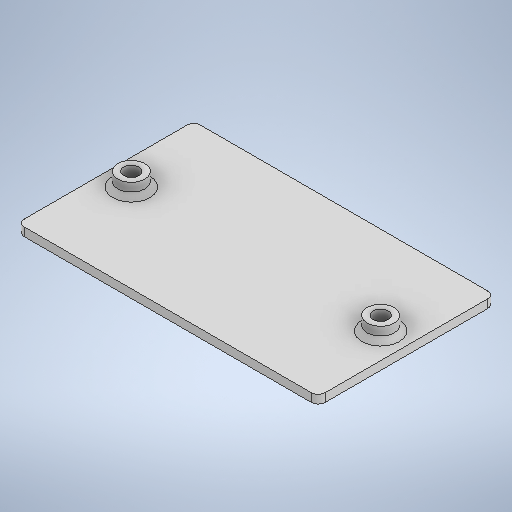
# Autodesk Inventor part: medium_backplate
Saved by Autodesk Inventor 2025.2 (Build 292293000, 293)
## iProperties
Created: 2025-04-21
Part Number: medium_backplate
Material: Generic
Document SubType Name: Modeling
Designer: osmon
Density: 1 g/cm^3
Appearance: Default
Author: osmon
Autodesk Inventor part; units mm, degrees
ref_plane "YZ Plane" through (0, 0, 0) normal (1, 0, 0) x (0, 1, 0)
ref_plane "XZ Plane" through (0, 0, 0) normal (0, 1, 0) x (-1, 0, 0)
ref_plane "XY Plane" through (0, 0, 0) normal (0, 0, 1) x (1, 0, 0)
sketch "Sketch1" plane through (0, 0, 0) normal (0, 1, 0) x (-1, 0, 0)
  line L0 (0, 0) -> (-88.9, 0)
  line L1 (-88.9, 0) -> (-88.9, -52.1)
  line L2 (-88.9, -52.1) -> (0, -52.1)
  line L3 (0, -52.1) -> (0, 0)
  dimension "d0" = 88.9
  dimension "d1" = 52.1
  constraints: 8 end point, 2 parallel, 1 horizontal, 1 perpendicular
  measures "d0" distance of L2.end L1.end
  measures "d1" distance of L1.end L0.end
extrude "Extrusion1" add sketch "Sketch1" along normal blind 2.5
sketch "Sketch2" plane through (0, 2.5, 0) normal (0, 1, 0) x (1, 0, 0)
  circle A0 centre (7.6, 26.05) radius 4
  circle A1 centre (81.3, 26.05) radius 4
  line L0 (0, 52.1) -> (0, 0) projected
  line L1 (88.9, 0) -> (88.9, 52.1) projected
  line L2 (88.9, 52.1) -> (0, 52.1) projected
  dimension "d4" = 8
  dimension "d5" = 8
  dimension "d6" = 7.6
  dimension "d7" = 7.6
  dimension "d8" = 26.05
  dimension "d9" = 26.05
  constraints: 2 centre point
  measures "d4" diameter of A0
  measures "d5" diameter of A1
  measures "d6" distance from line of L0 A0.centre
  measures "d7" distance from line of L1 A1.centre
  measures "d8" distance from line of L2 A0.centre
  measures "d9" distance from line of L2 A1.centre
extrude "Extrusion2" add sketch "Sketch2" along normal blind 4
sketch "Sketch3" plane through (7.6, 6.5, -26.05) normal (0, 1, 0) x (1, 0, 0)
  circle A0 centre (0, 0) radius 4 projected
  circle A1 centre (73.7, 0) radius 4 projected
  circle A2 centre (0, 0) radius 2.25
  circle A3 centre (73.7, 0) radius 2.25
  point P0 (-7.6, -26.05)
  dimension "d12" = 4.5
  dimension "d13" = 4.5
  constraints: 2 centre point, 2 coincident
  measures "d12" diameter of A2
  measures "d13" diameter of A3
extrude "Extrusion3" cut sketch "Sketch3" against normal blind 4.2 contours A2 | A3
chamfer "Chamfer1" distance 1.5 angle 45 2 edges at (77.3, 2.5, -26.05) (3.6, 2.5, -26.05)
fillet "Fillet1" radius 2 4 edges at (0, 1.25, 0) (88.9, 1.25, 0) (88.9, 1.25, -52.1) (0, 1.25, -52.1)
body "Solid1"
